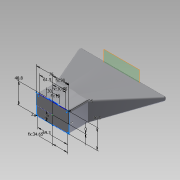
# Autodesk Inventor part: Canon Flash Difuser 02
Saved by Autodesk Inventor 2012 (Build 160160000, 160)
## iProperties
Created: 2013-01-03
Part Number: Canon Flash Difuser 02
Material: Default
Document SubType Name: Modeling
Designer: ericchu
Density: 1 g/cm^3
Author: ericchu
Autodesk Inventor part; units mm, degrees
ref_plane "YZ Plane" through (0, 0, 0) normal (1, 0, 0) x (0, 1, 0)
ref_plane "XY Plane" through (0, 0, 0) normal (0, 0, 1) x (1, 0, 0)
sketch "Sketch2" plane through (0, 0, 0) normal (0, 1, 0) x (-1, 0, 0)
  line L0 (-30.75, 26.5) -> (30.75, 26.5) construction
  line L1 (-34.65, -20) -> (34.65, -20) construction
  line L2 (-38, 0) -> (38, 0) construction
  line L3 (-15, 28.8) -> (15, 28.8) construction
  line L4 (33, 26.5) -> (-33, 26.5)
  line L5 (-38, 21.5) -> (-38, -18)
  line L6 (-36, -20) -> (36, -20)
  line L7 (38, -18) -> (38, 21.5)
  arc A0 (15, 26.5) -> (-15, 26.5) centre (0, -21.263) ccw
  arc A1 (-33, 26.5) -> (-38, 21.5) centre (-33, 21.5) ccw
  arc A2 (38, 21.5) -> (33, 26.5) centre (33, 21.5) ccw
  arc A3 (36, -20) -> (38, -18) centre (36, -18) ccw
  arc A4 (-38, -18) -> (-36, -20) centre (-36, -18) ccw
  point P0 (0, 0)
  point P1 (38, 26.5)
  point P2 (-38, -20)
  point P3 (-38, 26.5)
  point P4 (38, -20)
  dimension "d0" = 46.5
  dimension "d1" = 76
  dimension "d2" = 38
  dimension "d3" = 0
  dimension "d4" = 20
  dimension "d5" = 69.3
  dimension "d6" = 34.65
  dimension "d7" = 61.5
  dimension "d8" = 30.75
  dimension "d9" = 30
  dimension "d10" = 48.8
  dimension "d11" = 15
  dimension "d14" = 5
  dimension "d15" = 2
  constraints: 16 end point, 11 point on line, 10 point on circle, 8 tangent, 5 centre point, 5 parallel, 2 equal radius, 2 horizontal, 1 perpendicular
  measures "d0" distance between parallel lines of L1 L0
  measures "d1" distance of L2.start L2.end
  measures "d2" distance of point (0, 0) L2.start
  measures "d3" distance from line of point (0, 0) L2
  measures "d4" distance between parallel lines of L2 L1
  measures "d5" distance of L1.start L1.end
  measures "d6" horizontal distance of point (0, 0) L1.start
  measures "d7" distance of L0.start L0.end
  measures "d8" horizontal distance of point (0, 0) L0.start
  measures "d9" distance of L3.start L3.end
  measures "d10" distance between parallel lines of L1 L3
  measures "d11" horizontal distance of point (0, 0) L3.start
  measures "d14" radius of A1
  measures "d15" radius of A3
extrude "Extrusion1" add sketch "Sketch2" along normal blind 45
sketch "Sketch3" plane through (-38, 0, -18) normal (-1, 0, 0) x (0, 0, 1)
  line L0 (0, 0) -> (39.5, 0) projected
  line L1 (19.5, 8.5) -> (19.5, 3.5)
  line L2 (16.5, 3.5) -> (16.5, 8.5)
  arc A0 (16.5, 3.5) -> (19.5, 3.5) centre (18, 3.5) ccw
  arc A1 (19.5, 8.5) -> (16.5, 8.5) centre (18, 8.5) ccw
  line L3 (18, 10) -> (18, 2)
  point P0 (18, 0)
  dimension "d16" = 3
  dimension "d17" = 5
  dimension "d18" = 1.5
  dimension "d19" = 2
  constraints: 6 end point, 6 point on circle, 2 centre point, 1 parallel
  measures "d16" distance of L1.end L2.start
  measures "d17" distance of L1.start L1.end
  measures "d18" distance from line of L2 point (18, 0)
  measures "d19" distance edge to line of A0 L0
revolve "Revolution1" cut sketch "Sketch3" angle 360 about axis through (-38, 10, 0) along (0, -1, 0) contours L1 A0 L3 A1
mirror "Mirror1" about plane through (0, 0, 0) normal (1, 0, 0) of "Revolution1"
ref_plane "Work Plane1" through (0, 162, 0) normal (0, 1, 0) x (-1, 0, 0)
sketch "Sketch4" plane through (0, 162, 0) normal (0, 1, 0) x (-1, 0, 0)
  line L0 (-97, 5) -> (97, 5)
  line L1 (100, 2) -> (100, -2)
  line L2 (97, -5) -> (-97, -5)
  line L3 (-100, -2) -> (-100, 2)
  arc A0 (-97, 5) -> (-100, 2) centre (-97, 2) ccw
  arc A1 (-100, -2) -> (-97, -5) centre (-97, -2) ccw
  arc A2 (100, 2) -> (97, 5) centre (97, 2) ccw
  arc A3 (97, -5) -> (100, -2) centre (97, -2) ccw
  point P0 (0, 0)
  point P1 (-100, 5)
  point P2 (100, -5)
  point P3 (100, 5)
  point P4 (-100, -5)
  dimension "d22" = 10
  dimension "d23" = 5
  dimension "d24" = 200
  dimension "d25" = 100
  dimension "d30" = 3
  constraints: 8 end point, 8 point on circle, 8 point on line, 8 tangent, 4 centre point, 3 equal radius, 2 parallel, 1 horizontal, 1 perpendicular
  measures "d22" distance between parallel lines of L2 L0
  measures "d23" distance from line of point (0, 0) L2
  measures "d24" distance between parallel lines of L1 L3
  measures "d25" distance from line of point (0, 0) L3
  measures "d30" radius of A0
loft "Loft1" add profiles "Sketch4" section 1 edges at (0, 45, 28.8) (24, 45, 26.5) (36.5355, 45, 25.0355) (38, 45, 1.75) (37.4142, 45, -19.4142) (0, 45, -20) (-37.4142, 45, -19.4142) (-38, 45, 1.75) (-36.5355, 45, 25.0355) (-24, 45, 26.5)
sketch "Sketch5" plane through (-97, 162, -5) normal (0, 1, 0) x (1, 0, 0)
  line L0 (197, -7) -> (197, -3) projected
  arc A0 (197, -3) -> (194, 0) centre (194, -3) ccw projected
  line L1 (194, 0) -> (0, 0) projected
  arc A1 (0, 0) -> (-3, -3) centre (0, -3) ccw projected
  line L2 (-3, -3) -> (-3, -7) projected
  line L3 (-3, -5) -> (197, -5)
  point P0 (97, -5)
  constraints: 2 end point, 2 midpoint
revolve "Revolution2" add sketch "Sketch5" angle 180 about axis through (-100, 162, 0) along (1, 0, 0)
equation "\"d2\" = 0.5 * d1"
equation "\"d6\" = 0.5 * d5"
equation "\"d8\" = 0.5 * d7"
equation "\"d11\" = 0.5 * d9"
equation "\"d18\" = 0.5 * d16"
equation "\"d23\" = 0.5 * d22"
equation "\"d25\" = 0.5 * d24"
body "Solid1"
